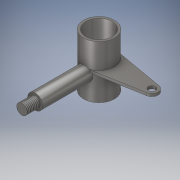
# Autodesk Inventor part: steering_kingpin
Saved by Autodesk Inventor 2019 (Build 230136000, 136)
## iProperties
Created: 2019-04-24
Part Number: steering_kingpin
Material: Steel, Mild
Document SubType Name: Modeling
Designer: callum.snowden
Density: 7.85 g/cm^3
Appearance: Semi-Polished
Mass: 256.931 g
Surface Area: 187.315 cm^2
Volume: 32.7301 cm^3
Author: callum.snowden
Autodesk Inventor part; units mm, degrees
sketch "Sketch1" plane through (0, 0, 0) normal (0, 1, 0) x (-1, 0, 0)
  line L0 (0, -24.5) -> (0, 24.5) construction
  line L1 (-24.5, 0) -> (24.5, 0) construction
  circle A0 centre (0, 0) radius 17.5
  circle A1 centre (0, 0) radius 15
  dimension "d0" = 35
  dimension "d1" = 30
  constraints: 2 centre point, 2 coincident
  measures "d0" diameter of A0
  measures "d1" diameter of A1
extrude "Extrusion1" add sketch "Sketch1" along normal blind 60
ref_plane "Work Plane4" through (0, 0, 17.5) normal (0, 0, 1) x (1, 0, 0)
sketch "Sketch2" plane through (0, 0, 17.5) normal (0, 0, 1) x (1, 0, 0)
  line L0 (17.5, 60) -> (-17.5, 60) construction
  line L1 (-17.5, 0) -> (17.5, 0) construction
  line L2 (0, 84) -> (0, -14) construction
  circle A0 centre (0, 25) radius 8.5
  point P0 (0, 0)
  dimension "d5" = 17
  dimension "d6" = 25
  constraints: 1 centre point, 1 point on line
  measures "d5" diameter of A0
  measures "d6" distance from line of L1 A0.centre
extrude "Extrusion2" add sketch "Sketch2" along normal blind 55
extrude "Extrusion3" add sketch "Sketch2" against normal up to next
sketch "Sketch3" plane through (0, 25, 72.5) normal (0, 0, 1) x (1, 0, 0)
  circle A0 centre (0, 0) radius 8.5 construction
  circle A1 centre (0, 0) radius 6
  point P0 (0, -25)
  dimension "d11" = 12
  constraints: 1 centre point, 1 coincident
  measures "d11" diameter of A1
extrude "Extrusion4" add sketch "Sketch3" along normal blind 15
thread "Thread1" size "M12x1.75" class "6g" standard "ISO Metric profile" length 15
ref_plane "Work Plane5" through (17.5, 0, 0) normal (1, 0, 0) x (0, 1, 0)
ref_plane "Work Plane6" through (0, 30, 0) normal (0, -1, 0) x (1, 0, 0)
sketch "Sketch7" plane through (0, 30, 0) normal (0, -1, 0) x (1, 0, 0)
  circle A0 centre (0, 0) radius 15 construction
  line L0 (0, 24.5) -> (0, -24.5) construction
  line L1 (-34.4, 0) -> (83.9, 0) construction
  arc A1 (61.225, -6.892) -> (61.225, 6.892) centre (60, 0) ccw
  line L2 (3.0625, -17.2299) -> (61.225, -6.892)
  line L3 (3.0625, 17.2299) -> (61.225, 6.892)
  arc A2 (3.0625, -17.2299) -> (3.0625, 17.2299) centre (0, 0) ccw
  circle A3 centre (60, 0) radius 4
  dimension "d35" = 14
  dimension "d36" = 60
  dimension "d37" = 8
  constraints: 4 centre point, 4 end point, 4 point on circle, 4 tangent, 1 coincident, 1 point on line
  measures "d35" diameter of A1
  measures "d36" distance of A1.centre point (0, 0)
  measures "d37" diameter of A3
extrude "Extrusion5" add sketch "Sketch7" along normal mid plane 3
equation "\"d23\" = 55deg"
equation "\"Sketch4_Pitch\" = 1.75"
body "Solid1"
